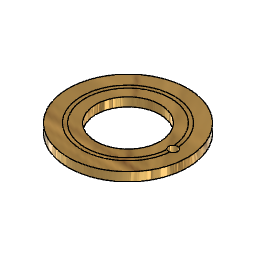
Engine Block Layer Plywood v4 (Autodesk Fusion 360 design; units mm, degrees)
Autodesk Fusion 360 part; units mm, degrees
note: some values were not read from the file. Set by a fixed rule: which face or edge a step refers to.
sketch "Sketch1" plane through (0, 0, 0) normal (0, 0, 1) x (1, 0, 0)
  circle A0 centre (17.385, 5) radius 11
  circle A1 centre (17.385, 5) radius 20.5
  circle A2 centre (32.885, 5) radius 1.55
  dimension "d3" = 22
  dimension "d4" = 41
  dimension "d9" = 3.1
  measures "d3" diameter of A0
  measures "d4" diameter of A1
  measures "d9" diameter of A2
extrude "Extrude1" add sketch "Sketch1" along normal blind 3
sketch "Sketch2" plane through (0, 0, 3) normal (0, 0, 1) x (-1, 0, 0)
  circle A0 centre (-17.385, -5) radius 11
  circle A1 centre (-17.385, -5) radius 20.5
  circle A2 centre (-17.385, -5) radius 14.65
  circle A3 centre (-17.385, -5) radius 15.9
  circle A4 centre (-32.885, -5) radius 1.55
  dimension "d7" = 29.3
  dimension "d8" = 31.8
  constraint concentric A0 A2
  constraint concentric A2 A3
  measures "d7" diameter of A2
  measures "d8" diameter of A3
split_face "SplitFace1" 1 faces at (31.8969, -0.0595, 3) by curves path "Sketch2" along A3
split_face "SplitFace2" 1 faces at (30.8785, 7.7452, 3) by curves path "Sketch2" along A2
